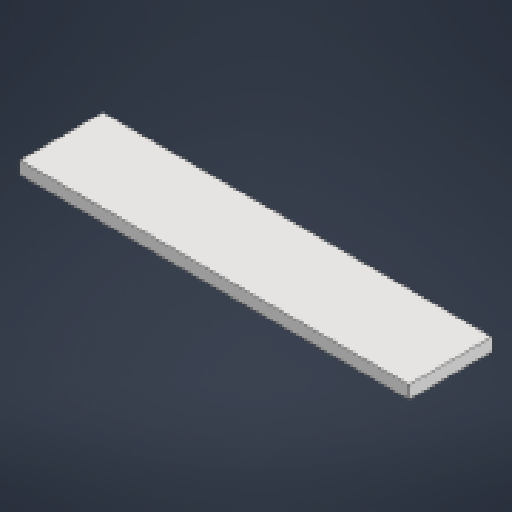
# Autodesk Inventor part: Parallel_Spacer
Saved by Autodesk Inventor 2024.3 (Build 283343000, 343)
## iProperties
Created: 2024-08-21
Part Number: Parallel_Spacer
Material: Generic
Document SubType Name: Modeling
Designer: fablabadmin
Density: 1 g/cm^3
Appearance: Default
Author: fablabadmin
Autodesk Inventor part; units mm, degrees
ref_plane "YZ Plane" through (0, 0, 0) normal (1, 0, 0) x (0, 1, 0)
ref_plane "XZ Plane" through (0, 0, 0) normal (0, 1, 0) x (-1, 0, 0)
ref_plane "XY Plane" through (0, 0, 0) normal (0, 0, 1) x (1, 0, 0)
sketch "Sketch1" plane through (0, 0, 0) normal (0, 1, 0) x (-1, 0, 0)
  line L0 (-75, 15.875) -> (75, 15.875)
  line L1 (75, 15.875) -> (75, -15.875)
  line L2 (75, -15.875) -> (-75, -15.875)
  line L3 (-75, -15.875) -> (-75, 15.875)
  line L4 (-75, 15.875) -> (75, -15.875) construction
  line L5 (75, 15.875) -> (-75, -15.875) construction
  point P0 (0, 0)
  dimension "d0" = 150
  dimension "d1" = 31.75
  constraints: 12 end point, 2 midpoint, 2 parallel, 1 horizontal, 1 perpendicular
  measures "d0" distance of L1.end L2.end
  measures "d1" distance of L0.end L1.end
extrude "Extrusion1" add sketch "Sketch1" along normal mid plane 4.7
body "Solid1"
